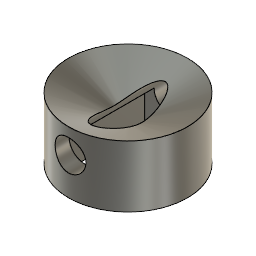
cat-dispenser-body-fusion (Autodesk Fusion 360 design; units mm, degrees)
Autodesk Fusion 360 part; units mm, degrees
sketch "Esboço1" plane through (0, 0, 0) normal (1, 0, 0) x (0, 1, 0)
  line L0 (0, 0) -> (48.25, 0)
  line L1 (48.25, 0) -> (48.25, 50)
  line L2 (48.25, 50) -> (0, 30)
  line L3 (0, 30) -> (0, 0)
  constraint coincident L0.start L3.end
  constraint horizontal L0
  constraint perpendicular L0 L1
  constraint perpendicular L0 L3
revolve "Revolucionar1" add sketch "Esboço1" angle 360 about axis through (0, 0, 30) along (0, 0, -1)
sketch "Esboço2" plane through (0, 0, 0) normal (0, 1, 0) x (1, 0, 0)
  circle A0 centre (0, -30) radius 12.5
  dimension "d3" = 25
  measures "d3" diameter of A0
extrude "Extrusão1" cut sketch "Esboço2" against normal blind 100
sketch "Esboço3" plane through (0, 0, 0) normal (0, -1, 0) x (1, 0, 0)
  line L0 (11.5473, 34.7864) -> (0, 30)
  line L1 (0, 30) -> (-11.5473, 34.7864)
  arc A0 (-11.5473, 34.7864) -> (11.5473, 34.7864) centre (0, 30) ccw
extrude "Extrusão2" cut sketch "Esboço3" against normal blind 100
sketch "Esboço4" plane through (0, 0, 0) normal (1, 0, 0) x (0, 1, 0)
sketch "Esboço5" plane through (0, 0, 0) normal (0, 1, 0) x (1, 0, 0)
  circle A0 centre (0, -30) radius 12.5
  dimension "d8" = 25
  measures "d8" diameter of A0
extrude "Extrusão3" cut sketch "Esboço5" along normal blind 50
sketch "Esboço6" plane through (0, 0, 0) normal (1, 0, 0) x (0, 1, 0)
sketch "Esboço7" plane through (0, 0, 0) normal (0, 1, 0) x (1, 0, 0)
sketch "Esboço8" plane through (0, 0, 0) normal (0, 0, -1) x (1, 0, 0)
  circle A0 centre (0, 0) radius 48.25
  line L0 (-20.1188, 35.2904) -> (20.1188, 35.2904)
  line L1 (20.1188, 35.2904) -> (20.1188, -33.6413)
  line L2 (20.1188, -33.6413) -> (-20.1188, -33.6413)
  line L3 (-20.1188, -33.6413) -> (-20.1188, 35.2904)
  constraint horizontal L0
  constraint vertical L1
  constraint horizontal L2
  constraint vertical L3
extrude "Extrusão4" cut sketch "Esboço8" against normal blind 30 contours L0 L1 L2 L3
